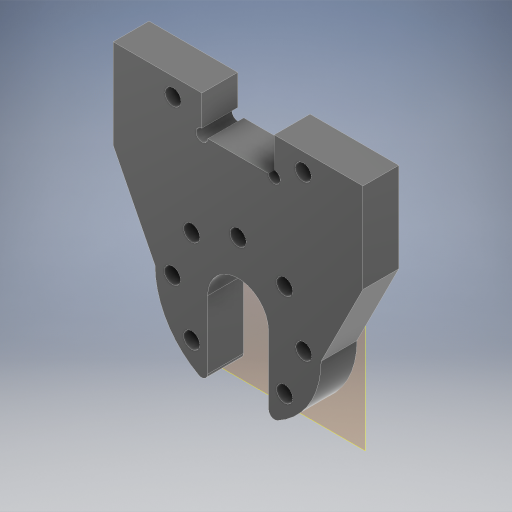
# Autodesk Inventor part: leg_between_64
Saved by Autodesk Inventor 2024 (Build 280153000, 153)
## iProperties
Created: 2024-09-03
Part Number: leg_between_64
Material: PMMA 플라스틱
Document SubType Name: Modeling
Designer: msi
Density: 1.188 g/cm^3
Appearance: 매끄러움 - 검은색
Author: msi
Autodesk Inventor part; units mm, degrees
ref_plane "YZ Plane" through (0, 0, 0) normal (1, 0, 0) x (0, 1, 0)
ref_plane "XZ Plane" through (0, 0, 0) normal (0, 1, 0) x (-1, 0, 0)
ref_plane "XY Plane" through (0, 0, 0) normal (0, 0, 1) x (1, 0, 0)
ref_plane "작업 평면1" through (0, 0, 0) normal (0, 0, 1) x (1, 0, 0)
sketch "스케치1" plane through (0, 0, 0) normal (0, 0, 1) x (1, 0, 0)
  circle A0 centre (-7.7782, -7.7782) radius 1.55 projected
  circle A1 centre (7.7782, -7.7782) radius 1.55 projected
  circle A2 centre (7.7782, 7.7782) radius 1.55 projected
  circle A3 centre (-7.7782, 7.7782) radius 1.55 projected
  circle A4 centre (0, 0) radius 5 projected
  circle A5 centre (0, 0) radius 13.9 projected
  circle A6 centre (0, 11) radius 1.55 projected
  circle A7 centre (11, 0) radius 1.55 projected
  circle A8 centre (0, -11) radius 1.55 projected
  circle A9 centre (-11, 0) radius 1.55 projected
  line L0 (13.9, 0) -> (13.9, 13.9)
  line L1 (13.9, 13.9) -> (-13.9, 13.9)
  line L2 (-13.9, 13.9) -> (13.9, 13.9)
  line L3 (13.9, 28.9) -> (-13.9, 28.9)
  line L4 (3.1, 28.9) -> (-3.1, 28.9)
  circle A10 centre (0, 0) radius 5.1
  circle A11 centre (-7.7782, 7.7782) radius 1.35
  circle A12 centre (-11, 0) radius 1.35
  circle A13 centre (-7.7782, -7.7782) radius 1.35
  circle A14 centre (0, -11) radius 1.35
  circle A15 centre (7.7782, -7.7782) radius 1.35
  circle A16 centre (11, 0) radius 1.35
  circle A17 centre (7.7782, 7.7782) radius 1.35
  circle A18 centre (0, 11) radius 1.35
  circle A19 centre (0, 0) radius 13.9
  line L5 (-5.1, 0) -> (-5.1, -12.9306)
  line L6 (5.1, 0) -> (5.1, -12.9306)
  line L7 (6.05, 28.9) -> (-6.05, 28.9)
  line L8 (-6.05, 28.9) -> (-6.05, 22.8)
  line L9 (-6.05, 22.8) -> (6.05, 22.8)
  line L10 (6.05, 22.8) -> (6.05, 28.9)
  line L11 (13.9, 28.9) -> (20.9, 28.9)
  line L12 (20.9, 28.9) -> (20.9, 13.9)
  line L13 (20.9, 13.9) -> (13.9, 13.9)
  line L14 (-13.9, 28.9) -> (-20.9, 28.9)
  line L15 (-20.9, 28.9) -> (-20.9, 13.9)
  line L16 (-20.9, 13.9) -> (-13.9, 13.9)
  line L17 (-20.9, 13.9) -> (-13.9, 0)
  line L18 (13.9, 0) -> (20.9, 13.9)
  circle A20 centre (-10.9, 25.9) radius 1.35
  circle A21 centre (10.9, 25.9) radius 1.35
  point P0 (0, 0)
  point P1 (0, 13.9)
  dimension "d24" = 0.1
  dimension "d25" = 2.7
  dimension "d28" = 360
  dimension "d30" = 12.1
  dimension "d31" = 6.1
  dimension "d39" = 2.7
  dimension "d40" = 2.7
  constraints: 38 end point, 12 centre point, 6 point on circle, 5 horizontal, 5 parallel, 3 perpendicular, 3 point on line, 2 coincident, 1 tangent, 1 vertical, 20 other
  measures "d24" radial gap between concentric circles of A4 A10
  measures "d25" diameter of A11
  measures "d30" distance of L9.end L8.end
  measures "d31" distance of L8.end L7.end
  measures "d39" diameter of A20
  measures "d40" diameter of A21
extrude "돌출7" add sketch "스케치1" along normal blind 6 contours A0 | A1 | A2 | A3 | A5 L6 A10 L5 | L17 L16 L1 A5 | L1 L0 A5 | L1 L16 L15 L14 L3 L8 L9 L10 L11 L12 L13 | L0 L13 L18 | A6 | A7 | A9 picked at (-7.5104, -2.4224)
fillet "모깎기3" radius 1 2 edges at (-5.1, -12.9306, 3) (5.1, -12.9306, 3)
sketch "스케치2" plane through (0, 0, 6) normal (0, 0, 1) x (1, 0, 0)
  line L0 (-6.05, 22.8) -> (-6.05, 28.9) projected
  line L1 (6.05, 22.8) -> (-6.05, 22.8) projected
  line L2 (6.05, 28.9) -> (6.05, 22.8) projected
  circle A0 centre (-6.05, 22.8) radius 1
  circle A1 centre (6.05, 22.8) radius 1
  point P0 (0, 0)
  dimension "d47" = 2
  dimension "d48" = 2
  constraints: 2 centre point, 2 coincident
  measures "d47" diameter of A0
  measures "d48" diameter of A1
extrude "돌출8" cut sketch "스케치2" against normal blind 10
